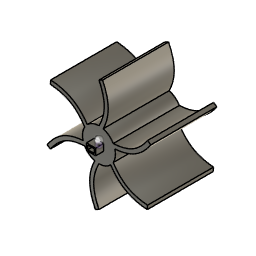
HELICE v2 (Autodesk Fusion 360 design; units mm, degrees)
Autodesk Fusion 360 part; units mm, degrees
sketch "Boceto1" plane through (0, 0, 0) normal (0, 1, 0) x (1, 0, 0)
  circle A0 centre (0, 0) radius 12.5
  spline S0 degree 5 poles (0.0283, -12.5) (0.331, -13.0785) (0.9099, -14.2374) (1.6984, -15.9815) (2.5873, -18.3184) (3.4097, -21.2601) (3.9181, -24.224) (4.0879, -27.2119) (3.9073, -30.2248) (3.3923, -33.2613) (2.5689, -36.3197) (1.6843, -38.7825) (0.9018, -40.638) (0.3281, -41.8787) (0.0283, -42.5) knots 0 0 0 0 0 0 0.1 0.2 0.3 0.4 0.5 0.6 0.7 0.8 0.9 1 1 1 1 1 1
  spline S1 degree 5 poles (10.8394, -6.2255) (11.4918, -6.2526) (12.7849, -6.3307) (14.6896, -6.5199) (17.1579, -6.9185) (20.1166, -7.6771) (22.9377, -8.7188) (25.6102, -10.0658) (28.1291, -11.7286) (30.5013, -13.6929) (32.7383, -15.9351) (34.4288, -17.9326) (35.6444, -19.538) (36.4321, -20.6552) (36.8202, -21.2255) knots 0 0 0 0 0 0 0.1 0.2 0.3 0.4 0.5 0.6 0.7 0.8 0.9 1 1 1 1 1 1
  spline S2 degree 5 poles (10.8112, 6.2745) (11.1608, 6.8259) (11.875, 7.9067) (12.9912, 9.4616) (14.5705, 11.3999) (16.7069, 13.5829) (19.0195, 15.5052) (21.5223, 17.1462) (24.2218, 18.4962) (27.109, 19.5684) (30.1693, 20.3846) (32.7445, 20.8499) (34.7427, 21.1) (36.104, 21.2235) (36.7919, 21.2745) knots 0 0 0 0 0 0 0.1 0.2 0.3 0.4 0.5 0.6 0.7 0.8 0.9 1 1 1 1 1 1
  spline S3 degree 5 poles (-0.0283, 12.5) (-0.331, 13.0785) (-0.9099, 14.2374) (-1.6984, 15.9815) (-2.5873, 18.3184) (-3.4097, 21.2601) (-3.9181, 24.224) (-4.0879, 27.2119) (-3.9073, 30.2248) (-3.3923, 33.2613) (-2.5689, 36.3197) (-1.6843, 38.7825) (-0.9018, 40.638) (-0.3281, 41.8787) (-0.0283, 42.5) knots 0 0 0 0 0 0 0.1 0.2 0.3 0.4 0.5 0.6 0.7 0.8 0.9 1 1 1 1 1 1
  spline S4 degree 5 poles (-10.8394, 6.2255) (-11.4918, 6.2526) (-12.7849, 6.3307) (-14.6896, 6.5199) (-17.1579, 6.9185) (-20.1166, 7.6771) (-22.9377, 8.7188) (-25.6102, 10.0658) (-28.1291, 11.7286) (-30.5013, 13.6929) (-32.7383, 15.9351) (-34.4288, 17.9326) (-35.6444, 19.538) (-36.4321, 20.6552) (-36.8202, 21.2255) knots 0 0 0 0 0 0 0.1 0.2 0.3 0.4 0.5 0.6 0.7 0.8 0.9 1 1 1 1 1 1
  spline S5 degree 5 poles (-10.8112, -6.2745) (-11.1608, -6.8259) (-11.875, -7.9067) (-12.9912, -9.4616) (-14.5705, -11.3999) (-16.7069, -13.5829) (-19.0195, -15.5052) (-21.5223, -17.1462) (-24.2218, -18.4962) (-27.109, -19.5684) (-30.1693, -20.3846) (-32.7445, -20.8499) (-34.7427, -21.1) (-36.104, -21.2235) (-36.7919, -21.2745) knots 0 0 0 0 0 0 0.1 0.2 0.3 0.4 0.5 0.6 0.7 0.8 0.9 1 1 1 1 1 1
  spline S6 degree 3 poles (2.6863, -11.1089) (4.8889, -15.3178) (6.376, -19.6566) (6.8447, -24.1702) (7.2296, -27.8773) (6.8659, -31.6563) (5.8959, -35.3638) (5.1552, -38.1952) (4.0833, -41.0001) (2.7301, -43.8039) knots 0 0 0 0 0.408399 0.408399 0.408399 0.743829 0.743829 0.743829 1 1 1 1
  spline S7 degree 3 poles (10.9638, -3.2281) (15.7101, -3.425) (20.2111, -4.3065) (24.3543, -6.1574) (27.7573, -7.6776) (30.8481, -9.8821) (33.5739, -12.5759) (35.6556, -14.6331) (37.5487, -16.9638) (39.3004, -19.5377) knots 0 0 0 0 0.408399 0.408399 0.408399 0.743829 0.743829 0.743829 1 1 1 1
  spline S8 degree 3 poles (8.2775, 7.8809) (10.8212, 11.8928) (13.8351, 15.3501) (17.5096, 18.0128) (20.5276, 20.1997) (23.9822, 21.7741) (27.678, 22.7879) (30.5004, 23.5621) (33.4655, 24.0362) (36.5703, 24.2663) knots 0 0 0 0 0.408399 0.408399 0.408399 0.743829 0.743829 0.743829 1 1 1 1
  spline S9 degree 3 poles (-2.6863, 11.1089) (-4.8889, 15.3178) (-6.376, 19.6566) (-6.8447, 24.1702) (-7.2296, 27.8773) (-6.8659, 31.6563) (-5.8959, 35.3638) (-5.1552, 38.1952) (-4.0833, 41.0001) (-2.7301, 43.8039) knots 0 0 0 0 0.408399 0.408399 0.408399 0.743829 0.743829 0.743829 1 1 1 1
  spline S10 degree 3 poles (-10.9638, 3.2281) (-15.7101, 3.425) (-20.2111, 4.3065) (-24.3543, 6.1574) (-27.7573, 7.6776) (-30.8481, 9.8821) (-33.5739, 12.5759) (-35.6556, 14.6331) (-37.5487, 16.9638) (-39.3004, 19.5377) knots 0 0 0 0 0.408399 0.408399 0.408399 0.743829 0.743829 0.743829 1 1 1 1
  spline S11 degree 3 poles (-8.2775, -7.8809) (-10.8212, -11.8928) (-13.8351, -15.3501) (-17.5096, -18.0128) (-20.5276, -20.1997) (-23.9822, -21.7741) (-27.678, -22.7879) (-30.5004, -23.5621) (-33.4655, -24.0362) (-36.5703, -24.2663) knots 0 0 0 0 0.408399 0.408399 0.408399 0.743829 0.743829 0.743829 1 1 1 1
  line L0 (0.0283, -42.5) -> (2.7301, -43.8039)
  line L1 (36.8202, -21.2255) -> (39.3004, -19.5377)
  line L2 (-36.5703, -24.2663) -> (-36.7919, -21.2745)
  line L3 (-39.3004, 19.5377) -> (-36.8202, 21.2255)
  line L4 (-2.7301, 43.8039) -> (-0.0283, 42.5)
  line L5 (36.5703, 24.2663) -> (36.7919, 21.2745)
  point P0 (4, -27)
  point P1 (25.3827, -10.0359)
  point P2 (21.3827, 16.9641)
  point P3 (-4, 27)
  point P4 (-25.3827, 10.0359)
  point P5 (-21.3827, -16.9641)
  dimension "d1" = 25
  dimension "d5" = -3
  constraint coincident A0.centre origin
  constraint coincident A0 S0.start
  constraint parallel L1 L3
  constraint parallel L2 L5
  measures "d1" diameter of A0
extrude "Extruir1" add sketch "Boceto1" along normal blind 50
sketch "Boceto2" plane through (0, 0, 0) normal (0, -1, 0) x (1, 0, 0)
  arc A0 (-0.0283, -12.5) -> (8.8761, -8.8014) centre (0, 0) ccw
  spline S0 degree 3 poles (8.8761, -8.8014) (11.2912, -12.4227) (14.1192, -15.556) (17.5096, -18.0128) (20.5276, -20.1997) (23.9822, -21.7741) (27.678, -22.7879) (30.5004, -23.5621) (33.4655, -24.0362) (36.5703, -24.2663) knots 0.031578 0.031578 0.031578 0.031578 0.408399 0.408399 0.408399 0.743829 0.743829 0.743829 1 1 1 1
  line L0 (36.5703, -24.2663) -> (36.7919, -21.2745)
  spline S1 degree 5 poles (10.8112, -6.2745) (11.1608, -6.8259) (11.875, -7.9067) (12.9912, -9.4616) (14.5705, -11.3999) (16.7069, -13.5829) (19.0195, -15.5052) (21.5223, -17.1462) (24.2218, -18.4962) (27.109, -19.5684) (30.1693, -20.3846) (32.7445, -20.8499) (34.7427, -21.1) (36.104, -21.2235) (36.7919, -21.2745) knots 0 0 0 0 0 0 0.1 0.2 0.3 0.4 0.5 0.6 0.7 0.8 0.9 1 1 1 1 1 1
  arc A1 (10.8112, -6.2745) -> (12.0603, 3.2862) centre (0, 0) ccw
  spline S2 degree 3 poles (12.0603, 3.2862) (16.404, 3.5671) (20.5315, 4.4496) (24.3543, 6.1574) (27.7573, 7.6776) (30.8481, 9.8821) (33.5739, 12.5759) (35.6556, 14.6331) (37.5487, 16.9638) (39.3004, 19.5377) knots 0.031578 0.031578 0.031578 0.031578 0.408399 0.408399 0.408399 0.743829 0.743829 0.743829 1 1 1 1
  line L1 (39.3004, 19.5377) -> (36.8202, 21.2255)
  spline S3 degree 5 poles (10.8394, 6.2255) (11.4918, 6.2526) (12.7849, 6.3307) (14.6896, 6.5199) (17.1579, 6.9185) (20.1166, 7.6771) (22.9377, 8.7188) (25.6102, 10.0658) (28.1291, 11.7286) (30.5013, 13.6929) (32.7383, 15.9351) (34.4288, 17.9326) (35.6444, 19.538) (36.4321, 20.6552) (36.8202, 21.2255) knots 0 0 0 0 0 0 0.1 0.2 0.3 0.4 0.5 0.6 0.7 0.8 0.9 1 1 1 1 1 1
  arc A2 (10.8394, 6.2255) -> (3.1842, 12.0876) centre (0, 0) ccw
  spline S4 degree 3 poles (3.1842, 12.0876) (5.1128, 15.9898) (6.4123, 20.0056) (6.8447, 24.1702) (7.2296, 27.8773) (6.8659, 31.6563) (5.8959, 35.3638) (5.1552, 38.1952) (4.0833, 41.0001) (2.7301, 43.8039) knots 0.031578 0.031578 0.031578 0.031578 0.408399 0.408399 0.408399 0.743829 0.743829 0.743829 1 1 1 1
  line L2 (2.7301, 43.8039) -> (0.0283, 42.5)
  spline S5 degree 5 poles (0.0283, 12.5) (0.331, 13.0785) (0.9099, 14.2374) (1.6984, 15.9815) (2.5873, 18.3184) (3.4097, 21.2601) (3.9181, 24.224) (4.0879, 27.2119) (3.9073, 30.2248) (3.3923, 33.2613) (2.5689, 36.3197) (1.6843, 38.7825) (0.9018, 40.638) (0.3281, 41.8787) (0.0283, 42.5) knots 0 0 0 0 0 0 0.1 0.2 0.3 0.4 0.5 0.6 0.7 0.8 0.9 1 1 1 1 1 1
  arc A3 (0.0283, 12.5) -> (-8.8761, 8.8014) centre (0, 0) ccw
  spline S6 degree 3 poles (-8.8761, 8.8014) (-11.2912, 12.4227) (-14.1192, 15.556) (-17.5096, 18.0128) (-20.5276, 20.1997) (-23.9822, 21.7741) (-27.678, 22.7879) (-30.5004, 23.5621) (-33.4655, 24.0362) (-36.5703, 24.2663) knots 0.031578 0.031578 0.031578 0.031578 0.408399 0.408399 0.408399 0.743829 0.743829 0.743829 1 1 1 1
  line L3 (-36.5703, 24.2663) -> (-36.7919, 21.2745)
  spline S7 degree 5 poles (-10.8112, 6.2745) (-11.1608, 6.8259) (-11.875, 7.9067) (-12.9912, 9.4616) (-14.5705, 11.3999) (-16.7069, 13.5829) (-19.0195, 15.5052) (-21.5223, 17.1462) (-24.2218, 18.4962) (-27.109, 19.5684) (-30.1693, 20.3846) (-32.7445, 20.8499) (-34.7427, 21.1) (-36.104, 21.2235) (-36.7919, 21.2745) knots 0 0 0 0 0 0 0.1 0.2 0.3 0.4 0.5 0.6 0.7 0.8 0.9 1 1 1 1 1 1
  arc A4 (-10.8112, 6.2745) -> (-12.0603, -3.2862) centre (0, 0) ccw
  spline S8 degree 3 poles (-12.0603, -3.2862) (-16.404, -3.5671) (-20.5315, -4.4496) (-24.3543, -6.1574) (-27.7573, -7.6776) (-30.8481, -9.8821) (-33.5739, -12.5759) (-35.6556, -14.6331) (-37.5487, -16.9638) (-39.3004, -19.5377) knots 0.031578 0.031578 0.031578 0.031578 0.408399 0.408399 0.408399 0.743829 0.743829 0.743829 1 1 1 1
  line L4 (-39.3004, -19.5377) -> (-36.8202, -21.2255)
  spline S9 degree 5 poles (-10.8394, -6.2255) (-11.4918, -6.2526) (-12.7849, -6.3307) (-14.6896, -6.5199) (-17.1579, -6.9185) (-20.1166, -7.6771) (-22.9377, -8.7188) (-25.6102, -10.0658) (-28.1291, -11.7286) (-30.5013, -13.6929) (-32.7383, -15.9351) (-34.4288, -17.9326) (-35.6444, -19.538) (-36.4321, -20.6552) (-36.8202, -21.2255) knots 0 0 0 0 0 0 0.1 0.2 0.3 0.4 0.5 0.6 0.7 0.8 0.9 1 1 1 1 1 1
  arc A5 (-10.8394, -6.2255) -> (-3.1842, -12.0876) centre (0, 0) ccw
  spline S10 degree 3 poles (-3.1842, -12.0876) (-5.1128, -15.9898) (-6.4123, -20.0056) (-6.8447, -24.1702) (-7.2296, -27.8773) (-6.8659, -31.6563) (-5.8959, -35.3638) (-5.1552, -38.1952) (-4.0833, -41.0001) (-2.7301, -43.8039) knots 0.031578 0.031578 0.031578 0.031578 0.408399 0.408399 0.408399 0.743829 0.743829 0.743829 1 1 1 1
  line L5 (-2.7301, -43.8039) -> (-0.0283, -42.5)
  spline S11 degree 5 poles (-0.0283, -12.5) (-0.331, -13.0785) (-0.9099, -14.2374) (-1.6984, -15.9815) (-2.5873, -18.3184) (-3.4097, -21.2601) (-3.9181, -24.224) (-4.0879, -27.2119) (-3.9073, -30.2248) (-3.3923, -33.2613) (-2.5689, -36.3197) (-1.6843, -38.7825) (-0.9018, -40.638) (-0.3281, -41.8787) (-0.0283, -42.5) knots 0 0 0 0 0 0 0.1 0.2 0.3 0.4 0.5 0.6 0.7 0.8 0.9 1 1 1 1 1 1
  line L6 (0, 0) -> (-2.5, 0)
  line L7 (-2.5, 0) -> (-2.5, 1.5)
  line L8 (-2.5, 1.5) -> (2.5, 1.5)
  line L9 (2.5, 1.5) -> (2.5, -1.5)
  line L10 (2.5, -1.5) -> (-2.5, -1.5)
  line L11 (-2.5, -1.5) -> (-2.5, 0)
  line L12 (-3.5, -2.5) -> (-3.5, 2.5)
  line L13 (-3.5, 2.5) -> (3.5, 2.5)
  line L14 (3.5, 2.5) -> (3.5, -2.5)
  line L15 (3.5, -2.5) -> (-3.5, -2.5)
  dimension "d10" = 2.5
  dimension "d11" = 1.5
  dimension "d12" = 5
  dimension "d13" = 3
  constraint coincident A0.centre A1.centre
  constraint horizontal L6
  constraint perpendicular L6 L7
  constraint perpendicular L7 L8
  constraint perpendicular L8 L9
  constraint perpendicular L7 L10
  constraint perpendicular L6 L11
  constraint perpendicular L12 L13
  constraint perpendicular L13 L14
  measures "d10" distance of A0.centre L6.end
  measures "d11" distance of L6.end L7.end
  measures "d12" distance of L7.end L8.end
  measures "d13" distance of L8.end L9.end
extrude "Extruir2" add sketch "Boceto2" along normal blind 6 contours L12 L13 L14 L15
sketch "Boceto3" plane through (0, 0, 0) normal (0, 1, 0) x (1, 0, 0)
  line L0 (0, 0) -> (0, -2.9052)
  constraint coincident L0.start origin
  constraint vertical L0
